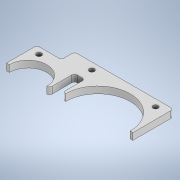
# Autodesk Inventor part: Bottle layout pt3
Saved by Autodesk Inventor 2021 (Build 250183000, 183)
## iProperties
Created: 2020-07-28
Part Number: Bottle layout pt3
Material: Generic
Document SubType Name: Modeling
Designer: jgray
Density: 1 g/cm^3
Appearance: Default
Author: jgray
Autodesk Inventor part; units mm, degrees
ref_plane "YZ Plane" through (0, 0, 0) normal (1, 0, 0) x (0, 1, 0)
ref_plane "XZ Plane" through (0, 0, 0) normal (0, 1, 0) x (-1, 0, 0)
ref_plane "XY Plane" through (0, 0, 0) normal (0, 0, 1) x (1, 0, 0)
sketch "Sketch1" plane through (0, 0, 0) normal (0, 1, 0) x (-1, 0, 0)
  line L0 (-56.25, 58.25) -> (56.25, 58.25)
  line L1 (56.25, 58.25) -> (56.25, -58.25)
  line L2 (56.25, -58.25) -> (-56.25, -58.25)
  line L3 (-56.25, -58.25) -> (-56.25, 58.25)
  line L4 (-56.25, 58.25) -> (56.25, -58.25) construction
  line L5 (56.25, 58.25) -> (-56.25, -58.25) construction
  point P0 (0, 0)
  dimension "d0" = 112.5
  dimension "d1" = 116.5
  constraints: 12 end point, 2 midpoint, 2 parallel, 1 horizontal, 1 perpendicular
  measures "d0" distance of L1.end L2.end
  measures "d1" distance of L0.end L1.end
extrude "Extrusion1" add sketch "Sketch1" along normal blind 5
sketch "Sketch2" plane through (0, 5, 0) normal (0, 1, 0) x (1, 0, 0)
  circle A0 centre (18.5, 28) radius 23.85
  circle A1 centre (37, -23.25) radius 13.85
  circle A2 centre (-35, -40.25) radius 13.85
  circle A3 centre (-30.9, 25.8) radius 13.85
  circle A4 centre (0, -23.25) radius 13.85
  line L0 (56.25, 58.25) -> (-56.25, 58.25) projected
  line L1 (-56.25, -58.25) -> (56.25, -58.25) projected
  line L2 (0, -105.9299) -> (0, 123.2086) construction
  line L3 (-76.4777, -40.25) -> (-5.35, -40.25) construction
  line L4 (-123.5447, -23.25) -> (82.5572, -23.25) construction
  line L5 (56.25, -58.25) -> (56.25, 58.25) construction
  point P0 (0, 0)
  dimension "d4" = 47.7
  dimension "d5" = 27.7
  dimension "d6" = 27.7
  dimension "d7" = 27.7
  dimension "d8" = 27.7
  dimension "d9" = 116.5
  dimension "d10" = 112.5
  dimension "d13" = 37
  dimension "d14" = 18.5
  dimension "d15" = 30.9
  dimension "d18" = 18
  dimension "d19" = 35
  dimension "d20" = 35
  dimension "d93" = 25.8
  dimension "d94" = 28
  constraints: 6 end point, 5 centre point, 5 point on line, 1 horizontal, 1 perpendicular, 1 vertical
  measures "d4" diameter of A0
  measures "d5" diameter of A1
  measures "d6" diameter of A2
  measures "d7" diameter of A3
  measures "d8" diameter of A4
  measures "d9" distance between parallel lines of L0 L1
  measures "d10" distance of L1.start L1.end
  measures "d13" distance of A4.centre A1.centre
  measures "d14" distance from line of A0.centre L2
  measures "d15" distance from line of A3.centre L2
  measures "d18" distance between parallel lines of L1 L3
  measures "d19" distance between parallel lines of L1 L4
  measures "d20" horizontal distance of A2.centre A4.centre
  measures "d93" vertical distance of point (0, 0) A3.centre
  measures "d94" vertical distance of point (0, 0) A0.centre
extrude "Extrusion2" cut sketch "Sketch2" against normal blind 5
sketch "Sketch4" plane through (0, 5, 0) normal (0, 1, 0) x (1, 0, 0)
  line L0 (-56.25, 58.25) -> (-56.25, -58.25) construction
  circle A0 centre (0, -23.25) radius 13.85 construction
  circle A1 centre (37, -23.25) radius 13.85 construction
  circle A2 centre (-30.9, 25.8) radius 13.85 construction
  line L1 (56.25, 58.25) -> (-56.25, 58.25) construction
  line L2 (-17.15, -23.25) -> (-13.85, -23.25) construction
  line L3 (-46.75, -8.1822) -> (-46.85, -8.1822)
  line L4 (-13.85, -23.25) -> (-17.15, -23.25)
  line L5 (56.25, -58.25) -> (56.25, 58.25)
  line L6 (-46.85, -8.1822) -> (-46.75, -8.1822)
  arc A3 (-13.85, -23.25) -> (13.85, -23.25) centre (0, -23.25) ccw
  arc A4 (23.15, -23.25) -> (50.85, -23.25) centre (37, -23.25) ccw
  line L7 (-44.75, 58.25) -> (42.35, 58.25)
  line L8 (-48.85, -40.25) -> (-48.85, -40.25)
  line L9 (-50.85, -38.25) -> (-50.85, -10.1822)
  line L10 (-48.85, -8.1822) -> (-48.75, -8.1822)
  arc A5 (-50.85, -38.25) -> (-48.85, -40.25) centre (-48.85, -38.25) ccw
  arc A6 (-48.85, -8.1822) -> (-50.85, -10.1822) centre (-48.85, -10.1822) ccw
  line L11 (50.85, -23.25) -> (50.85, -23.25)
  line L12 (52.85, -21.25) -> (52.85, -4.75)
  line L13 (50.85, -2.75) -> (46.35, -2.75)
  arc A7 (50.85, -23.25) -> (52.85, -21.25) centre (50.85, -21.25) ccw
  arc A8 (52.85, -4.75) -> (50.85, -2.75) centre (50.85, -4.75) ccw
  line L14 (-44.7516, 25.8) -> (-44.7516, 25.8)
  line L15 (-46.75, 28.0339) -> (-46.75, 58.25)
  line L16 (-44.75, 58.25) -> (-46.75, 58.25)
  line L17 (-17.0566, 26.2282) -> (-17.0566, 26.2282)
  line L18 (-15.05, 27.8) -> (-15.05, 42.25)
  line L19 (-5.35, 27.98) -> (-5.35, 27.98)
  line L20 (-7.35, 29.9796) -> (-7.35, 42.25)
  line L21 (42.35, 27.98) -> (42.35, 27.98)
  line L22 (44.35, 58.25) -> (42.35, 58.25)
  circle A9 centre (0, -23.25) radius 13.85
  circle A10 centre (37, -23.25) radius 13.85
  line L23 (44.35, 58.25) -> (44.35, -0.75)
  line L24 (42.35, 27.98) -> (44.35, 27.98)
  line L25 (-5.35, 27.98) -> (-5.35, 27.98)
  line L26 (-7.35, 29.98) -> (-7.35, 29.9796)
  line L27 (-17.0566, 26.2282) -> (-17.0566, 26.2282)
  line L28 (-15.05, 28.0029) -> (-15.05, 28.0029)
  line L29 (-46.75, 28.0339) -> (-46.75, -6.1822)
  arc A11 (-48.75, -8.1822) -> (-46.75, -6.1822) centre (-48.75, -6.1822) ccw
  line L30 (-44.75, 25.8) -> (-46.75, 25.8)
  line L31 (-21.15, -40.25) -> (-21.15, -40.25)
  line L32 (-19.15, -38.25) -> (-19.15, -25.25)
  arc A12 (-21.15, -40.25) -> (-19.15, -38.25) centre (-21.15, -38.25) ccw
  arc A13 (-17.15, -23.25) -> (-19.15, -25.25) centre (-17.15, -25.25) ccw
  line L33 (-17.05, 25.8) -> (-17.05, 25.8)
  arc A14 (-17.05, 25.8) -> (-15.05, 27.8) centre (-17.05, 27.8) ccw
  line L34 (-56.25, -58.25) -> (56.25, -58.25)
  line L35 (56.25, -58.25) -> (56.25, 58.25)
  line L36 (56.25, 58.25) -> (-56.25, 58.25)
  line L37 (-56.25, 58.25) -> (-56.25, -58.25)
  circle A15 centre (-30.9, 25.8) radius 13.85
  circle A16 centre (-30.9, 25.8) radius 13.85
  line L38 (13.85, -23.25) -> (13.85, -13.25)
  circle A17 centre (0, -23.25) radius 13.85
  line L39 (23.15, -23.25) -> (23.15, -13.25)
  circle A18 centre (37, -23.25) radius 13.85
  arc A19 (23.15, -13.25) -> (13.85, -13.25) centre (18.5, -13.25) ccw
  circle A20 centre (18.5, 28) radius 23.85
  circle A21 centre (18.5, 28) radius 23.85
  line L40 (56.25, 58.25) -> (-56.25, 58.25)
  circle A22 centre (-35, -40.25) radius 13.85
  circle A23 centre (-35, -40.25) radius 13.85
  arc A24 (44.35, -0.75) -> (46.35, -2.75) centre (46.35, -0.75) ccw
  line L41 (-5.35, 27.98) -> (-5.35, 27.98)
  arc A25 (-7.35, 29.98) -> (-5.35, 27.98) centre (-5.35, 29.98) ccw
  circle A26 centre (18.5, 28) radius 23.85 projected
  circle A27 centre (37, -23.25) radius 13.85 projected
  circle A28 centre (-30.9, 25.8) radius 13.85 projected
  circle A29 centre (0, -23.25) radius 13.85 projected
  circle A30 centre (-35, -40.25) radius 13.85 projected
  line L42 (56.25, 58.25) -> (-56.25, 58.25) projected
  line L43 (-56.25, 58.25) -> (-56.25, -58.25) projected
  line L44 (-56.25, -58.25) -> (56.25, -58.25) projected
  line L45 (56.25, -58.25) -> (56.25, 58.25) projected
  line L46 (-13.05, 44.25) -> (-9.35, 44.25)
  arc A31 (-13.05, 44.25) -> (-15.05, 42.25) centre (-13.05, 42.25) ccw
  arc A32 (-7.35, 42.25) -> (-9.35, 44.25) centre (-9.35, 42.25) ccw
  point P0 (50.85, -23.25)
  point P1 (46.35, -2.8696)
  point P2 (50.85, -23.25)
  point P3 (-21.15, -40.25)
  point P4 (-7.35, 29.9796)
  point P5 (-5.35, 27.9796)
  point P6 (42.35, 27.9796)
  point P7 (-7.35, 58.25)
  point P8 (50.85, -23.25)
  point P9 (-21.15, -40.25)
  point P10 (-44.75, 25.8313)
  point P11 (-17.05, 25.8198)
  point P12 (0, 0)
  point P13 (0, 0)
  point P14 (44.35, -2.75)
  point P15 (-15.05, 58.25)
  point P16 (-7.35, 58.25)
  point P17 (-50.85, -40.25)
  point P18 (52.85, -23.25)
  point P19 (50.85, -23.25)
  point P20 (50.85, -23.25)
  point P21 (-7.35, 58.25)
  point P22 (50.85, -23.25)
  point P23 (-17.05, 25.8)
  point P24 (-7.35, 27.98)
  point P25 (-7.35, 29.98)
  point P26 (-21.15, -40.25)
  point P27 (50.85, -23.25)
  point P28 (13.85, -23.25)
  point P29 (42.35, 28)
  point P30 (-7.35, 29.98)
  point P31 (-17.05, 25.8)
  point P32 (-5.35, 27.98)
  point P33 (42.35, 27.98)
  point P34 (42.35, 27.98)
  dimension "d70" = 27.7
  dimension "d71" = 27.7
  dimension "d54" = 2
  dimension "d55" = 2
  dimension "d56" = 2
  dimension "d57" = 2
  dimension "d58" = 2
  dimension "d59" = 2
  dimension "d60" = 2
  dimension "d61" = 2
  dimension "d62" = 2
  dimension "d63" = 27.7
  dimension "d64" = 10
  dimension "d65" = 10
  dimension "d66" = 25.8
  dimension "d67" = 23.25
  dimension "d68" = 23.25
  dimension "d69" = 37
  dimension "d72" = 19.15
  dimension "d73" = 50.85
  dimension "d74" = 46.75
  dimension "d75" = 2
  dimension "d76" = 6.1822
  dimension "d77" = 31.7
  dimension "d78" = 51.7
  dimension "d79" = 30.9
  dimension "d80" = 3.4
  dimension "d81" = 11.9
  dimension "d82" = 61
  dimension "d83" = 47.7
  dimension "d84" = 28
  dimension "d85" = 18.5
  dimension "d86" = 30.27
  dimension "d87" = 27.7
  dimension "d88" = 2
  dimension "d89" = 30.27
  dimension "d90" = 2
  dimension "d91" = 112.5
  dimension "d92" = 116.5
  dimension "d96" = 14
  dimension "d97" = 2
  constraints: 84 end point, 40 point on circle, 30 tangent, 25 centre point, 23 point on line, 16 perpendicular, 9 horizontal, 5 coincident, 5 vertical, 4 equal radius, 3 parallel, 2 collinear, 2 concentric, 1 horizontal alignment, 1 line through centre, 1 midpoint, 14 other
  measures "d54" distance of L8.start point (-50.85, -40.25)
  measures "d55" radius of A5
  measures "d56" distance of L11.start point (52.85, -23.25)
  measures "d57" radius of A7
  measures "d58" distance from line of L21.end L23
  measures "d59" radius of A11
  measures "d60" radius of A12
  measures "d61" distance from line of L18 L33.start
  measures "d62" radius of A14
  measures "d63" diameter of A2
  measures "d64" distance of L38.start L38.end
  measures "d65" distance of L39.start L39.end
  measures "d66" vertical distance of point (0, 0) A2.centre
  measures "d67" vertical distance of point (0, 0) A1.centre
  measures "d68" distance of point (0, 0) A0.centre
  measures "d69" horizontal distance of A1.centre point (0, 0)
  measures "d72" distance from line of L32 point (0, 0)
  measures "d73" distance from line of L9 point (0, 0)
  measures "d74" distance from line of L29 point (0, 0)
  measures "d75" radius of A6
  measures "d76" vertical distance of point (0, 0) A11.centre
  measures "d77" distance between parallel lines of L18 L15
  measures "d78" distance between parallel lines of L23 L20
  measures "d79" horizontal distance of point (0, 0) A15.centre
  measures "d80" distance between parallel lines of L5 L12
  measures "d81" distance between parallel lines of L5 L23
  measures "d82" distance between parallel lines of L1 L13
  measures "d83" diameter of A20
  measures "d84" vertical distance of point (0, 0) A21.centre
  measures "d85" horizontal distance of A21.centre point (0, 0)
  measures "d86" distance between parallel lines of L7 L24
  measures "d87" diameter of A22
  measures "d88" radius of A24
  measures "d89" distance of point (-7.35, 58.25) point (-7.35, 27.98)
  measures "d90" radius of A25
  measures "d91" distance between parallel lines of L35 L0
  measures "d92" distance between parallel lines of L36 L34
  measures "d96" distance between parallel lines of L1 L46
  measures "d97" radius of A31
extrude "Extrusion3" cut sketch "Sketch4" against normal blind 10 contours A3 L38 A19 L39 A4 A7 L12 A8 L13 A24 L23 L36 L5 L34 L37 L15 L29 A11 L10 A6 L9 A5 A22 A12 L32 A13 L4 | L4 A13 L32 A12 A22 A5 L9 A6 L10 A11 L29 L30 A15 A14 L18 A31 L46 A32 L20 A25 A20 L24 L23 A24 L13 A8 L12 A7 A10 L39 A19 L38 A9
sketch "Sketch5" plane through (0, 5, 0) normal (0, 1, 0) x (1, 0, 0)
  line L0 (56.25, 58.25) -> (-56.25, 58.25) projected
  line L1 (56.25, 58.25) -> (-56.25, 58.25) projected
  line L2 (-46.75, 25.8) -> (-44.75, 25.8) projected
  arc A0 (-17.05, 25.8) -> (-44.75, 25.8) centre (-30.9, 25.8) ccw projected
  arc A1 (-17.05, 25.8) -> (-15.05, 27.8) centre (-17.05, 27.8) ccw projected
  line L3 (-15.05, 27.8) -> (-15.05, 42.25) projected
  arc A2 (-13.05, 44.25) -> (-15.05, 42.25) centre (-13.05, 42.25) ccw projected
  line L4 (-13.05, 44.25) -> (-9.35, 44.25) projected
  arc A3 (-7.35, 42.25) -> (-9.35, 44.25) centre (-9.35, 42.25) ccw projected
  line L5 (-7.35, 42.25) -> (-7.35, 29.9796) projected
  arc A4 (-7.35, 29.9796) -> (-5.35, 27.98) centre (-5.35, 29.98) ccw projected
  arc A5 (42.35, 27.98) -> (-5.35, 27.98) centre (18.5, 28) ccw projected
  line L6 (42.35, 27.98) -> (44.35, 27.98) projected
  line L7 (44.35, 27.98) -> (44.35, 58.25) projected
  line L8 (44.35, 58.25) -> (-46.75, 58.25) projected
  line L9 (-46.75, 58.25) -> (-46.75, 25.8) projected
  point P0 (0, 0)
  point P1 (-40.25, 43.25)
  point P2 (-10.75, 52.75)
  point P3 (36.35, 52.75)
  dimension "d40" = 5.5
  dimension "d41" = 5.5
  dimension "d44" = 15
  dimension "d99" = 6.5
  dimension "d100" = 36
  dimension "d101" = 8
  measures "d40" distance from line of L0 point (36.35, 52.75)
  measures "d41" distance from line of L0 point (-10.75, 52.75)
  measures "d44" distance from line of L1 point (-40.25, 43.25)
  measures "d99" distance from line of point (-40.25, 43.25) L9
  measures "d100" distance from line of point (-10.75, 52.75) L9
  measures "d101" distance from line of point (36.35, 52.75) L7
hole "Hole1" at (-40.25, 5, -43.25) at (-10.75, 5, -52.75) at (36.35, 5, -52.75) direction (0, -1, 0) diameter 3.8 end through all
sketch "Sketch6" plane through (0, 5, 0) normal (0, 1, 0) x (1, 0, 0)
  line L0 (44.35, 58.25) -> (-46.75, 58.25) projected
  line L1 (-28.75, 58.25) -> (-46.75, 58.25)
  line L2 (-46.75, 58.25) -> (-46.75, 48.25)
  line L3 (-46.75, 48.25) -> (-28.75, 48.25)
  line L4 (-28.75, 48.25) -> (-28.75, 58.25)
  line L5 (-46.75, 58.25) -> (-46.75, 25.8) projected
  point P0 (0, 0)
  point P1 (42.35, 58.25)
  point P2 (-44.75, 58.25)
  point P3 (-46.75, 56.25)
  point P4 (-44.75, 58.25)
  dimension "d102" = 18
  dimension "d103" = 10
  constraints: 8 end point, 2 parallel, 1 collinear, 1 horizontal, 1 perpendicular, 1 point on line
  measures "d102" distance of L3.end L2.end
  measures "d103" distance of L2.end L0.end
extrude "Extrusion4" cut sketch "Sketch6" against normal blind 10
sketch "Sketch8" plane through (44.35, 0, -58.25) normal (0, 0, -1) x (-1, 0, 0)
  line L0 (0, 5) -> (73.1, 5) projected
  line L1 (0, 0) -> (73.1, 0) projected
  line L2 (73.1, 5) -> (0, 5)
  line L3 (0, 5) -> (0, 0)
  line L4 (0, 0) -> (73.1, 0)
  line L5 (73.1, 0) -> (73.1, 5)
  point P0 (44.35, 0)
  constraints: 8 end point, 2 parallel, 1 horizontal, 1 perpendicular
extrude "Extrusion6" cut sketch "Sketch8" against normal blind 0.3
fillet "Fillet3" radius 2 4 edges at (-28.75, 2.5, -48.25) (-28.75, 2.5, -57.95) (44.35, 2.5, -57.95) (-46.75, 2.5, -48.25)
body "Solid1"
